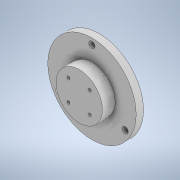
# Autodesk Inventor part: tampa traseira acoplada final
Saved by Autodesk Inventor 2022.1 (Build 261234020, 234B)
## iProperties
Created: 2023-08-18
Part Number: tampa traseira acoplada final
Material: Generic
Document SubType Name: Modeling
Designer: SENAI
Density: 1 g/cm^3
Appearance: Default
Author: SENAI
Autodesk Inventor part; units mm, degrees
ref_plane "YZ Plane" through (0, 0, 0) normal (1, 0, 0) x (0, 1, 0)
ref_plane "XZ Plane" through (0, 0, 0) normal (0, 1, 0) x (-1, 0, 0)
ref_plane "XY Plane" through (0, 0, 0) normal (0, 0, 1) x (1, 0, 0)
sketch "Sketch1" plane through (0, 0, 0) normal (0, 0, 1) x (1, 0, 0)
  circle A0 centre (0, 0) radius 60
  dimension "d0" = 120
  constraints: 1 centre point, 1 coincident
  measures "d0" diameter of A0
extrude "Extrusion1" add sketch "Sketch1" along normal blind 10
sketch "Sketch2" plane through (0, 0, 10) normal (0, 0, 1) x (1, 0, 0)
  circle A0 centre (0, 0) radius 31.5
  dimension "d3" = 63
  constraints: 1 centre point, 1 coincident
  measures "d3" diameter of A0
extrude "Extrusion2" add sketch "Sketch2" along normal blind 17.4
sketch "Sketch3" plane through (0, 0, 27.4) normal (0, 0, 1) x (1, 0, 0)
  circle A0 centre (-14.5, 14.5) radius 2
  circle A1 centre (14.5, 14.5) radius 2
  circle A2 centre (14.5, -14.5) radius 2
  circle A3 centre (-14.5, -14.5) radius 2
  point P0 (0, 0)
  dimension "d6" = 4
  dimension "d7" = 4
  dimension "d8" = 4
  dimension "d9" = 4
  dimension "d10" = 29
  dimension "d11" = 29
  dimension "d12" = 29
  dimension "d13" = 29
  dimension "d18" = 20.5061
  dimension "d19" = 20.5061
  dimension "d20" = 20.5061
  constraints: 4 centre point
  measures "d6" diameter of A0
  measures "d7" diameter of A1
  measures "d8" diameter of A2
  measures "d9" diameter of A3
  measures "d10" distance of A1.centre A0.centre
  measures "d11" distance of A2.centre A3.centre
  measures "d12" distance of A3.centre A0.centre
  measures "d13" distance of A2.centre A1.centre
  measures "d18" distance of point (0, 0) A1.centre
  measures "d19" distance of point (0, 0) A2.centre
  measures "d20" distance of point (0, 0) A0.centre
extrude "Extrusion3" cut sketch "Sketch3" against normal through all
sketch "Sketch4" plane through (0, 0, 0) normal (0, 0, -1) x (-1, 0, 0)
  circle A0 centre (0, 0) radius 44
  dimension "d23" = 88
  constraints: 1 centre point, 1 coincident
  measures "d23" diameter of A0
extrude "Extrusion4" add sketch "Sketch4" along normal blind 2
sketch "Sketch5" plane through (0, 0, -2) normal (0, 0, -1) x (-1, 0, 0)
  circle A0 centre (0, 0) radius 26
  dimension "d26" = 52
  constraints: 1 centre point, 1 coincident
  measures "d26" diameter of A0
extrude "Extrusion5" cut sketch "Sketch5" against normal blind 24
sketch "Sketch6" plane through (0, 0, 0) normal (0, 0, -1) x (-1, 0, 0)
  circle A0 centre (-45.068, -26.02) radius 4.2
  circle A1 centre (45.068, -26.02) radius 4.2
  circle A2 centre (0, 52) radius 4.2
  circle A3 centre (0, 0) radius 44 projected
  dimension "d29" = 8.4
  dimension "d30" = 8.4
  dimension "d31" = 8.4
  constraints: 3 centre point
  measures "d29" diameter of A0
  measures "d30" diameter of A1
  measures "d31" diameter of A2
extrude "Extrusion6" cut sketch "Sketch6" against normal blind 10 contours A0 | A1 | A2
body "Solid1"
